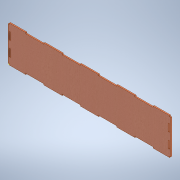
# Autodesk Inventor part: Lado superior
Saved by Autodesk Inventor 2020.3 (Build 243373000, 373)
## iProperties
Created: 2020-04-26
Part Number: Lado superior
Material: Madera (nogal)
Document SubType Name: Modeling
Designer: miosh
Density: 0.55 g/cm^3
Appearance: Nogal - Natural pulido
Author: miosh
Autodesk Inventor part; units mm, degrees
ref_plane "YZ Plane" through (0, 0, 0) normal (1, 0, 0) x (0, 1, 0)
ref_plane "XZ Plane" through (0, 0, 0) normal (0, 1, 0) x (-1, 0, 0)
ref_plane "XY Plane" through (0, 0, 0) normal (0, 0, 1) x (1, 0, 0)
sketch "Boceto1" plane through (0, 0, 0) normal (0, 0, 1) x (1, 0, 0)
  line L0 (3, 0) -> (3, 3)
  line L1 (3, 3) -> (0, 3)
  line L2 (0, 3) -> (0, 97)
  line L3 (0, 97) -> (3, 97)
  line L4 (3, 97) -> (3, 100)
  line L5 (3, 0) -> (48, 0)
  line L6 (48, 0) -> (48, 3)
  line L7 (48, 3) -> (98, 3)
  line L8 (98, 3) -> (98, 0)
  line L9 (98, 0) -> (148, 0)
  line L10 (148, 0) -> (148, 3)
  line L11 (148, 3) -> (198, 3)
  line L12 (198, 3) -> (198, 0)
  line L13 (198, 0) -> (248, 0)
  line L14 (248, 0) -> (248, 3)
  line L15 (248, 3) -> (298, 3)
  line L16 (298, 3) -> (298, 0)
  line L17 (298, 0) -> (348, 0)
  line L18 (348, 0) -> (348, 3)
  line L19 (348, 3) -> (398, 3)
  line L20 (398, 3) -> (398, 0)
  line L21 (398, 0) -> (443, 0)
  line L22 (443, 0) -> (443, 3)
  line L23 (443, 3) -> (446, 3)
  line L24 (446, 3) -> (446, 97)
  line L25 (446, 97) -> (443, 97)
  line L26 (443, 97) -> (443, 100)
  line L27 (443, 100) -> (398, 100)
  line L28 (398, 100) -> (398, 97)
  line L29 (398, 97) -> (348, 97)
  line L30 (348, 97) -> (348, 100)
  line L31 (348, 100) -> (298, 100)
  line L32 (298, 100) -> (298, 97)
  line L33 (298, 97) -> (248, 97)
  line L34 (248, 97) -> (248, 100)
  line L35 (248, 100) -> (198, 100)
  line L36 (198, 100) -> (198, 97)
  line L37 (198, 97) -> (148, 97)
  line L38 (148, 97) -> (148, 100)
  line L39 (148, 100) -> (98, 100)
  line L40 (98, 100) -> (98, 97)
  line L41 (98, 97) -> (48, 97)
  line L42 (48, 97) -> (48, 100)
  line L43 (48, 100) -> (3, 100)
  line L44 (3, 80) -> (6, 80)
  line L45 (6, 80) -> (6, 60)
  line L46 (6, 60) -> (3, 60)
  line L47 (3, 60) -> (3, 80)
  line L48 (3, 40) -> (6, 40)
  line L49 (6, 40) -> (6, 20)
  line L50 (6, 20) -> (3, 20)
  line L51 (3, 20) -> (3, 40)
  line L52 (443, 80) -> (440, 80)
  line L53 (440, 80) -> (440, 60)
  line L54 (440, 60) -> (443, 60)
  line L55 (443, 60) -> (443, 80)
  line L56 (443, 40) -> (440, 40)
  line L57 (440, 40) -> (440, 20)
  line L58 (440, 20) -> (443, 20)
  line L59 (443, 20) -> (443, 40)
  point P0 (0, 0)
  point P1 (3, 100)
  dimension "d0" = 3
  dimension "d1" = 94
  dimension "d2" = 3
  dimension "d3" = 3
  dimension "d4" = 45
  dimension "d5" = 3
  dimension "d6" = 50
  dimension "d7" = 3
  dimension "d8" = 50
  dimension "d9" = 3
  dimension "d10" = 50
  dimension "d11" = 3
  dimension "d12" = 50
  dimension "d13" = 3
  dimension "d14" = 50
  dimension "d15" = 3
  dimension "d16" = 50
  dimension "d17" = 3
  dimension "d18" = 50
  dimension "d19" = 3
  dimension "d20" = 45
  dimension "d21" = 3
  dimension "d22" = 3
  dimension "d23" = 94
  dimension "d41" = 3
  dimension "d42" = 45
  dimension "d43" = 3
  dimension "d44" = 50
  dimension "d45" = 3
  dimension "d46" = 50
  dimension "d58" = 3
  dimension "d59" = 50
  dimension "d60" = 3
  dimension "d61" = 50
  dimension "d62" = 3
  dimension "d63" = 50
  dimension "d64" = 3
  dimension "d65" = 50
  dimension "d66" = 3
  dimension "d67" = 50
  dimension "d68" = 3
  dimension "d71" = 20
  dimension "d72" = 3
  dimension "d73" = 20
  dimension "d75" = 20
  dimension "d76" = 3
  dimension "d77" = 20
  dimension "d78" = 3
  dimension "d79" = 20
  dimension "d80" = 3
  dimension "d81" = 20
  dimension "d82" = 20
  dimension "d83" = 3
  dimension "d84" = 20
  constraints: 120 end point, 26 perpendicular, 18 point on line, 6 vertical, 2 horizontal, 2 parallel
  measures "d0" distance of L0.start L0.end
  measures "d1" distance of L1.end L2.end
  measures "d2" distance of L2.end L3.end
  measures "d3" distance of L3.end L4.end
  measures "d4" distance of L0.start L5.end
  measures "d5" distance of L5.end L6.end
  measures "d6" distance of L6.end L7.end
  measures "d7" distance of L7.end L8.end
  measures "d8" distance of L8.end L9.end
  measures "d9" distance of L9.end L10.end
  measures "d10" distance of L10.end L11.end
  measures "d11" distance of L11.end L12.end
  measures "d12" distance of L12.end L13.end
  measures "d13" distance of L13.end L14.end
  measures "d14" distance of L14.end L15.end
  measures "d15" distance of L15.end L16.end
  measures "d16" distance of L16.end L17.end
  measures "d17" distance of L17.end L18.end
  measures "d18" distance of L18.end L19.end
  measures "d19" distance of L19.end L20.end
  measures "d20" distance of L20.end L21.end
  measures "d21" distance of L21.end L22.end
  measures "d22" distance of L22.end L23.end
  measures "d23" distance of L23.end L24.end
  measures "d41" distance of L25.end L26.end
  measures "d42" distance of L26.end L27.end
  measures "d43" distance of L27.end L28.end
  measures "d44" distance of L28.end L29.end
  measures "d45" distance of L29.end L30.end
  measures "d46" distance of L30.end L31.end
  measures "d58" distance of L31.end L32.end
  measures "d59" distance of L32.end L33.end
  measures "d60" distance of L33.end L34.end
  measures "d61" distance of L34.end L35.end
  measures "d62" distance of L35.end L36.end
  measures "d63" distance of L36.end L37.end
  measures "d64" distance of L37.end L38.end
  measures "d65" distance of L38.end L39.end
  measures "d66" distance of L39.end L40.end
  measures "d67" distance of L40.end L41.end
  measures "d68" distance of L41.end L42.end
  measures "d71" distance of L43.end L44.start
  measures "d72" distance of L44.start L44.end
  measures "d73" distance of L44.end L45.end
  measures "d75" distance of L46.end L48.start
  measures "d76" distance of L48.start L48.end
  measures "d77" distance of L48.end L49.end
  measures "d78" distance of L49.end L50.end
  measures "d79" distance of L26.end L52.start
  measures "d80" distance of L52.start L52.end
  measures "d81" distance of L52.end L53.end
  measures "d82" distance of L54.end L56.start
  measures "d83" distance of L56.start L56.end
  measures "d84" distance of L56.end L57.end
extrude "Extrusión1" add sketch "Boceto1" against normal blind 3 contours L0 L1 L2 L3 L4 L43 L42 L41 L40 L39 L38 L37 L36 L35 L34 L33 L32 L31 L30 L29 L28 L27 L26 L25 L24 L23 L22 L21 L20 L19 L18 L17 L16 L15 L14 L13 L12 L11 L10 L9 L8 L7 L6 L5 | L44 L45 L46 L47 | L48 L49 L50 L51 | L55 L54 L53 L52 | L59 L58 L57 L56
sketch "Boceto2" plane through (0, 0, -3) normal (0, 0, -1) x (1, 0, 0)
  point P0 (0, 0)
sketch "Boceto3" plane through (0, 0, 0) normal (0, 0, 1) x (1, 0, 0)
  line L0 (3, 97) -> (3, 100) projected
  line L1 (3, 80) -> (6, 80)
  line L2 (6, 80) -> (6, 60)
  line L3 (6, 60) -> (3, 60)
  line L4 (3, 60) -> (3, 80)
  line L5 (3, 40) -> (6, 40)
  line L6 (6, 40) -> (6, 20)
  line L7 (6, 20) -> (3, 20)
  line L8 (3, 20) -> (3, 40)
  line L9 (398, 100) -> (443, 100) projected
  line L10 (443, 80) -> (440, 80)
  line L11 (440, 80) -> (440, 60)
  line L12 (440, 60) -> (443, 60)
  line L13 (443, 60) -> (443, 80)
  line L14 (443, 40) -> (440, 40)
  line L15 (440, 40) -> (440, 20)
  line L16 (440, 20) -> (443, 20)
  line L17 (443, 20) -> (443, 40)
  point P0 (0, 0)
  dimension "d85" = 20
  dimension "d86" = 3
  dimension "d87" = 20
  dimension "d88" = 3
  dimension "d89" = 20
  dimension "d90" = 3
  dimension "d91" = 20
  dimension "d92" = 3
  dimension "d93" = 20
  dimension "d94" = 3
  dimension "d95" = 20
  dimension "d96" = 3
  dimension "d97" = 20
  dimension "d98" = 3
  dimension "d99" = 20
  dimension "d100" = 3
  constraints: 32 end point, 5 perpendicular, 1 parallel
  measures "d85" distance of L0.end L1.start
  measures "d86" distance of L1.start L1.end
  measures "d87" distance of L1.end L2.end
  measures "d88" distance of L2.end L3.end
  measures "d89" distance of L3.end L5.start
  measures "d90" distance of L5.start L5.end
  measures "d91" distance of L5.end L6.end
  measures "d92" distance of L6.end L7.end
  measures "d93" distance of L9.end L10.start
  measures "d94" distance of L10.start L10.end
  measures "d95" distance of L10.end L11.end
  measures "d96" distance of L11.end L12.end
  measures "d97" distance of L12.end L14.start
  measures "d98" distance of L14.start L14.end
  measures "d99" distance of L14.end L15.end
  measures "d100" distance of L15.end L16.end
extrude "Extrusión2" cut sketch "Boceto3" against normal blind 10
